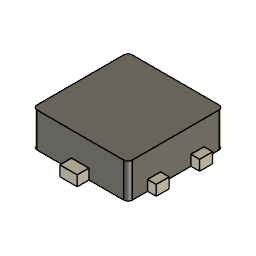
SKY13453-385LF (Autodesk Fusion 360 design; units mm, degrees)
Autodesk Fusion 360 part; units mm, degrees
sketch "草图1" plane through (0, 0, 0) normal (0, 0, 1) x (1, 0, 0)
  line L0 (0, 4) -> (0, -5) construction
  line L1 (-7.5, 0) -> (7.5, 0) construction
  line L2 (-0.1, 0.685) -> (0.1, 0.685)
  line L3 (0.1, 0.685) -> (0.1, 0.175)
  line L4 (0.1, 0.175) -> (-0.1, 0.175)
  line L5 (-0.1, 0.175) -> (-0.1, 0.685)
  line L6 (-0.1, -0.175) -> (0.1, -0.175)
  line L7 (0.1, -0.175) -> (0.1, -0.685)
  line L8 (0.1, -0.685) -> (-0.1, -0.685)
  line L9 (-0.1, -0.685) -> (-0.1, -0.175)
  line L10 (-0.32, 0.325) -> (-0.65, 0.325)
  line L11 (-0.65, 0.325) -> (-0.65, 0.175)
  line L12 (-0.65, 0.175) -> (-0.32, 0.175)
  line L13 (-0.32, 0.175) -> (-0.32, 0.325)
  line L14 (-0.65, -0.175) -> (-0.32, -0.175)
  line L15 (-0.32, -0.175) -> (-0.32, -0.325)
  line L16 (-0.32, -0.325) -> (-0.65, -0.325)
  line L17 (-0.65, -0.325) -> (-0.65, -0.175)
  line L18 (0.32, -0.325) -> (0.65, -0.325)
  line L19 (0.65, -0.175) -> (0.32, -0.175)
  line L20 (0.32, -0.175) -> (0.32, -0.325)
  line L21 (0.65, -0.325) -> (0.65, -0.175)
  line L22 (0.65, 0.325) -> (0.65, 0.175)
  line L23 (0.32, 0.325) -> (0.65, 0.325)
  line L24 (0.65, 0.175) -> (0.32, 0.175)
  line L25 (0.32, 0.175) -> (0.32, 0.325)
  line L26 (-0.5, 0.55) -> (0.5, 0.55)
  line L27 (0.55, 0.5) -> (0.55, -0.5)
  line L28 (0.5, -0.55) -> (-0.5, -0.55)
  line L29 (-0.55, -0.5) -> (-0.55, 0.5)
  arc A0 (-0.5, 0.55) -> (-0.55, 0.5) centre (-0.5, 0.5) ccw
  arc A1 (0.55, 0.5) -> (0.5, 0.55) centre (0.5, 0.5) ccw
  arc A2 (0.5, -0.55) -> (0.55, -0.5) centre (0.5, -0.5) ccw
  arc A3 (-0.55, -0.5) -> (-0.5, -0.55) centre (-0.5, -0.5) ccw
  dimension "d1" = 0.15
  dimension "d2" = 0.2
  dimension "d3" = 0.51
  dimension "d6" = 0.33
  dimension "d7" = 0.65
  dimension "d8" = 0.65
  dimension "d10" = 0.51
  dimension "d11" = 0.51
  dimension "d12" = 0.05
  dimension "d13" = 1
  dimension "d14" = 1
  constraint vertical L0
  constraint horizontal L1
  constraint horizontal L2
  constraint vertical L3
  constraint horizontal L4
  constraint vertical L5
  constraint horizontal L6
  constraint vertical L7
  constraint horizontal L8
  constraint vertical L9
  constraint horizontal L10
  constraint vertical L11
  constraint horizontal L12
  constraint vertical L13
  constraint horizontal L14
  constraint vertical L15
  constraint horizontal L16
  constraint vertical L17
  constraint equal L13 L17
  constraint equal L4 L8
  constraint symmetric L0 L3 L5
  constraint equal L3 L7
  constraint symmetric L1 L12 L14
  constraint equal L12 L14
  constraint collinear L11 L17
  constraint symmetric L0 L10.start L23.start
  constraint symmetric L0 L10.end L22.start
  constraint symmetric L0 L11.end L22.end
  constraint symmetric L0 L12.end L24.end
  constraint symmetric L0 L14.start L19.start
  constraint symmetric L0 L14.end L19.end
  constraint symmetric L0 L15.end L18.start
  constraint symmetric L0 L16.end L18.end
  constraint horizontal L26
  constraint vertical L27
  constraint horizontal L28
  constraint vertical L29
  constraint tangent L26 A0
  constraint tangent L29 A0
  constraint tangent L27 A1
  constraint tangent L26 A1
  constraint equal A0 A1
  constraint tangent L27 A2
  constraint tangent L28 A2
  constraint equal A0 A2
  constraint tangent L28 A3
  constraint tangent L29 A3
  constraint equal A0 A3
  constraint symmetric L1 L26 L28
  constraint symmetric L0 L27 L29
  measures "d1" distance of L10.start L12.end
  measures "d2" distance of L7.end L8.end
  measures "d3" distance of L2.end L3.end
  measures "d6" distance of L15.end L16.end
  measures "d7" distance of L10.end L16.end
  measures "d8" distance of L0 L10.end
  measures "d10" distance of L8 L19
  measures "d11" distance of L2 L24
  measures "d12" radius of A0
  measures "d13" distance of L26.start L26.end
  measures "d14" distance of L27.start L27.end
extrude "拉伸1" add sketch "草图1" along normal blind 0.4 contours L3 L4 L5 L26 | L3 L4 L5 L6 L7 L9 L10 L12 L13 L14 L15 L16 L18 L19 L20 L23 L24 L25 L26 L27 L28 L29 A0 A1 A2 A3 | L10 L12 L13 L29 | L23 L24 L25 L27 | L14 L15 L16 L29 | L18 L19 L20 L27 | L6 L7 L9 L28 makes body 1
extrude "拉伸2" cut sketch "草图1" along normal blind 0.12 contours L3 L4 L5 L26 | L10 L12 L13 L29 | L23 L24 L25 L27 | L14 L15 L16 L29 | L18 L19 L20 L27 | L6 L7 L9 L28 bodies 1
extrude "拉伸3" add sketch "草图1" along normal blind 0.12 separate body contours L2 L3 L5 L26 | L3 L4 L5 L26 | L10 L11 L12 L29 | L10 L12 L13 L29 | L23 L24 L25 L27 | L22 L23 L24 L27 | L14 L16 L17 L29 | L14 L15 L16 L29 | L18 L19 L20 L27 | L18 L19 L21 L27 | L7 L8 L9 L28 | L6 L7 L9 L28 makes body 2 at (0.0333, 0.345, 0) makes body 3 at (-0.0333, -0.345, 0) makes body 4 at (-0.54, 0.275, 0) makes body 5 at (0.54, 0.225, 0) makes body 6 at (0.43, -0.225, 0) makes body 7 at (-0.54, -0.225, 0)
